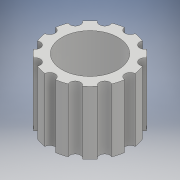
# Autodesk Inventor part: poulie 12 dents
Saved by Autodesk Inventor 2018.1 (Build 221171000, 171)
## iProperties
Created: 2022-05-13
Part Number: poulie 12 dents
Material: Generic
Document SubType Name: Modeling
Designer: Bureau
Density: 1 g/cm^3
Appearance: Default
Author: Bureau
Autodesk Inventor part; units mm, degrees
ref_plane "YZ Plane" through (0, 0, 0) normal (1, 0, 0) x (0, 1, 0)
ref_plane "XZ Plane" through (0, 0, 0) normal (0, 1, 0) x (-1, 0, 0)
ref_plane "XY Plane" through (0, 0, 0) normal (0, 0, 1) x (1, 0, 0)
sketch "Sketch1" plane through (0, 0, 0) normal (0, 0, 1) x (1, 0, 0)
  circle A0 centre (0, 0) radius 4
  arc A1 (-0.7484, 5.6809) -> (0.7484, 5.6809) centre (0, 5.73) ccw
  arc A2 (-3.4886, 4.5456) -> (-2.1923, 5.294) centre (-2.865, 4.9623) ccw
  arc A3 (-5.294, 2.1923) -> (-4.5456, 3.4886) centre (-4.9623, 2.865) ccw
  arc A4 (-5.6809, -0.7484) -> (-5.6809, 0.7484) centre (-5.73, 0) ccw
  arc A5 (-4.5456, -3.4886) -> (-5.294, -2.1923) centre (-4.9623, -2.865) ccw
  arc A6 (-2.1923, -5.294) -> (-3.4886, -4.5456) centre (-2.865, -4.9623) ccw
  arc A7 (0.7484, -5.6809) -> (-0.7484, -5.6809) centre (0, -5.73) ccw
  arc A8 (3.4886, -4.5456) -> (2.1923, -5.294) centre (2.865, -4.9623) ccw
  arc A9 (5.294, -2.1923) -> (4.5456, -3.4886) centre (4.9623, -2.865) ccw
  arc A10 (5.6809, 0.7484) -> (5.6809, -0.7484) centre (5.73, 0) ccw
  arc A11 (4.5456, 3.4886) -> (5.294, 2.1923) centre (4.9623, 2.865) ccw
  arc A12 (2.1923, 5.294) -> (3.4886, 4.5456) centre (2.865, 4.9623) ccw
  arc A13 (-0.7484, 5.6809) -> (-2.1923, 5.294) centre (0, 0) ccw
  arc A14 (-3.4886, 4.5456) -> (-4.5456, 3.4886) centre (0, 0) ccw
  arc A15 (-5.294, 2.1923) -> (-5.6809, 0.7484) centre (0, 0) ccw
  arc A16 (-5.6809, -0.7484) -> (-5.294, -2.1923) centre (0, 0) ccw
  arc A17 (2.1923, 5.294) -> (0.7484, 5.6809) centre (0, 0) ccw
  arc A18 (4.5456, 3.4886) -> (3.4886, 4.5456) centre (0, 0) ccw
  arc A19 (5.6809, 0.7484) -> (5.294, 2.1923) centre (0, 0) ccw
  arc A20 (5.294, -2.1923) -> (5.6809, -0.7484) centre (0, 0) ccw
  arc A21 (3.4886, -4.5456) -> (4.5456, -3.4886) centre (0, 0) ccw
  arc A22 (0.7484, -5.6809) -> (2.1923, -5.294) centre (0, 0) ccw
  arc A23 (-4.5456, -3.4886) -> (-3.4886, -4.5456) centre (0, 0) ccw
  arc A24 (-2.1923, -5.294) -> (-0.7484, -5.6809) centre (0, 0) ccw
  dimension "d0" = 8
  dimension "d2" = 1.5
  dimension "d5" = 360
  constraints: 48 point on circle, 25 centre point, 2 coincident, 49 other
  measures "d0" diameter of A0
  measures "d2" diameter of A1
extrude "Extrusion1" add sketch "Sketch1" along normal blind 9
body "Solid1"
